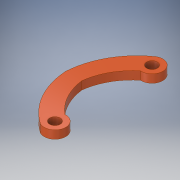
# Autodesk Inventor part: 000.703 - Тяга
Saved by Autodesk Inventor 2019 (Build 230136000, 136)
## iProperties
Created: 2020-02-29
Part Number: 000.703 - Тяга
Material: Пластик АБС
Document SubType Name: Modeling
Designer: Петров Иван
Density: 1.06 g/cm^3
Appearance: Гладкий — светло-оранжевый
Author: Петров Иван
Autodesk Inventor part; units mm, degrees
ref_plane "YZ Plane" through (0, 0, 0) normal (1, 0, 0) x (0, 1, 0)
ref_plane "XZ Plane" through (0, 0, 0) normal (0, 1, 0) x (-1, 0, 0)
ref_plane "XY Plane" through (0, 0, 0) normal (0, 0, 1) x (1, 0, 0)
sketch "Эскиз3" plane through (0, 0, 0) normal (0, 1, 0) x (-1, 0, 0)
  arc A0 (1.791, 3.5766) -> (0.2774, -3.9904) centre (0, 0) ccw
  arc A1 (14, -18) -> (1.791, 3.5766) centre (-14.1884, -19.7077) ccw
  arc A2 (8, -18) -> (0.2774, -3.9904) centre (-13.2839, -20.5991) ccw
  line L0 (8, -18) -> (14, -18)
  line L1 (0, 0) -> (13.752, 0)
  dimension "d12" = 8
  dimension "d27" = 8
  dimension "d29" = 18
  dimension "d30" = 6
  constraints: 8 point on circle, 4 end point, 3 centre point, 1 coincident, 1 horizontal, 1 parallel
  measures "d12" diameter of A0
  measures "d27" horizontal distance of L0.start point (0, 0)
  measures "d29" distance from line of point (0, 0) L0
  measures "d30" distance of L0.start L0.end
extrude "Выдавливание5" add sketch "Эскиз3" along normal blind 3
sketch "Эскиз5" plane through (0, 3, 0) normal (0, 1, 0) x (1, 0, 0)
  circle A0 centre (0, 0) radius 2
  dimension "d24" = 4
  constraints: 1 centre point, 1 coincident
  measures "d24" diameter of A0
extrude "Выдавливание6" cut sketch "Эскиз5" against normal blind 10
mirror "Зеркальное отражение1" about plane through (-8, 0, -18) normal (0, 0, -1) of "Выдавливание5", "Выдавливание6"
